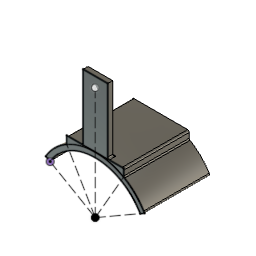
wriststrap v1 (Autodesk Fusion 360 design; units mm, degrees)
Autodesk Fusion 360 part; units mm, degrees
sketch "Sketch2" plane through (0, 0, 0) normal (0, 1, 0) x (1, 0, 0)
  arc A0 (0, 0) -> (55, 0) centre (27.5, 15.8771) ccw
  line L0 (0, 0) -> (27.5, 15.8771) construction
  line L1 (27.5, 15.8771) -> (55, 0) construction
  arc A1 (-2.5981, -1.5) -> (57.5981, -1.5) centre (27.5, 15.8771) ccw
  line L2 (0, 0) -> (-2.5981, -1.5)
  line L3 (57.5981, -1.5) -> (55, 0)
  line L4 (27.5, 15.8771) -> (27.5, -52.8095) construction
  line L5 (27.5, 15.8771) -> (10.1229, -14.2209) construction
  line L6 (27.5, 15.8771) -> (44.8771, -14.2209) construction
  line L7 (10.1229, -18.8771) -> (44.8771, -18.8771)
  line L8 (44.8771, -14.2209) -> (44.8771, -18.8771)
  line L9 (10.1229, -14.2209) -> (10.1229, -18.8771)
  line L10 (20.1229, -18.8771) -> (20.1229, -58.8771)
  line L11 (20.1229, -58.8771) -> (35.1229, -58.8771)
  line L12 (35.1229, -58.8771) -> (35.1229, -18.8771)
  dimension "d2" = 55
  dimension "d3" = 120
  dimension "d4" = 3
  dimension "d7" = 30
  dimension "d24" = 30
  dimension "d25" = 40
  dimension "d26" = 10
  dimension "d27" = 15
  constraint coincident A0.start L0.start
  constraint horizontal A0.start A0.end
  constraint coincident A0.centre L0.end
  constraint parallel L0 L2
  constraint parallel L1 L3
  constraint vertical L4
  constraint coincident A1 L5.end
  constraint coincident A1 L6.end
  constraint perpendicular L4 L7
  constraint tangent A1 L7
  constraint vertical L5.end L7.start
  constraint vertical L6.end L7.end
  constraint coincident L7 L10.start
  constraint perpendicular L7 L10
  constraint perpendicular L10 L11
  constraint coincident L7 L12.end
  constraint perpendicular L7 L12
  measures "d2" distance of A0.start A0.end
  measures "d3" angle of L0 L1
  measures "d7" angle of L4 L5
  measures "d24" angle of L4 L6
  measures "d25" distance of L7 L11
  measures "d26" distance of L9 L10
  measures "d27" distance of L10 L12
extrude "Extrude4" add sketch "Sketch2" along normal blind 40 contours A0 A1 L2 L3 | A1 L7 L9 | A1 L7 L8
extrude "Extrude5" add sketch "Sketch2" along normal blind 3 contours L7 L10 L11 L12
fillet "Fillet1" radius 1 7 edges at (10.1229, 20, 14.2209) (10.1229, 20, 18.8771) (44.8771, 20, 18.8771) (44.8771, 20, 14.2209) (27.6229, 3, 18.8771) (35.1229, 1.5, 18.8771) (20.1229, 1.5, 18.8771)
fillet "Fillet2" radius 1 4 edges at (57.5981, 20, 1.5) (55, 20, 0) (-2.5981, 20, 1.5) (0, 20, 0)
